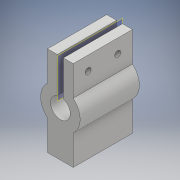
# Autodesk Inventor part: leverClamp
Saved by Autodesk Inventor 2018 (Build 220112000, 112)
## iProperties
Created: 2017-10-29
Part Number: leverClamp
Material: Generic
Document SubType Name: Modeling
Designer: Prakash
Density: 1 g/cm^3
Appearance: Default
Author: Prakash
Autodesk Inventor part; units mm, degrees
ref_plane "YZ Plane" through (0, 0, 0) normal (1, 0, 0) x (0, 1, 0)
ref_plane "XZ Plane" through (0, 0, 0) normal (0, 1, 0) x (-1, 0, 0)
ref_plane "XY Plane" through (0, 0, 0) normal (0, 0, 1) x (1, 0, 0)
sketch "Sketch1" plane through (0, 0, 0) normal (0, 1, 0) x (-1, 0, 0)
  arc A0 (5, -18) -> (5, -27.5394) centre (6.5, -22.7697) ccw
  line L0 (5, 0) -> (5, -18)
  line L1 (5, -27.5394) -> (5, -45.5394)
  line L2 (5, -18) -> (5, -27.5394) construction
  line L3 (5, -22.7697) -> (6.5, -22.7697) construction
  arc A1 (0, -15.1704) -> (0, -30.369) centre (6.5, -22.7697) ccw
  line L4 (0, 0) -> (0, -15.1704)
  line L5 (0, -30.369) -> (0, -45.5394)
  line L6 (5, 0) -> (0, 0)
  line L7 (0, -45.5394) -> (5, -45.5394)
  dimension "d0" = 10
  dimension "d1" = 1.5
  dimension "d2" = 5
  dimension "d4" = 5
  dimension "d5" = 18
  constraints: 16 end point, 5 point on circle, 3 coincident, 2 centre point, 2 collinear, 2 equal length, 2 horizontal, 2 vertical, 1 midpoint, 1 parallel
  measures "d0" diameter of A0
  measures "d1" distance of L3.start L3.end
  measures "d2" radial gap between concentric circles of A1 A0
  measures "d4" distance between parallel lines of L0 L4
  measures "d5" distance of L0.start L0.end
extrude "Extrusion1" add sketch "Sketch1" along normal blind 30
sketch "Sketch2" plane through (0, 0, 0) normal (1, 0, 0) x (0, 0, -1)
  line L0 (45.5394, 30) -> (27.5394, 30) projected
  line L1 (38.5394, 30) -> (38.5394, 0)
  line L2 (45.5394, 0) -> (45.5394, 30) projected
  line L3 (18, 30) -> (0, 30) projected
  line L4 (7, 30) -> (7, 0)
  line L5 (0, 0) -> (0, 30) projected
  line L6 (0, 0) -> (15.1704, 0) projected
  line L7 (30.369, 0) -> (45.5394, 0) projected
  point P0 (38.5394, 22.5)
  point P1 (38.5394, 7.5)
  point P2 (7, 22.5)
  point P3 (7, 7.5)
  dimension "d8" = 7
  dimension "d9" = 7
  dimension "d10" = 7.5
  dimension "d11" = 7.5
  dimension "d12" = 7.5
  dimension "d13" = 7.5
  dimension "d14" = 30
  dimension "d15" = 30
  constraints: 6 point on line, 4 end point, 2 vertical
  measures "d8" distance between parallel lines of L2 L1
  measures "d9" distance between parallel lines of L5 L4
  measures "d10" distance from line of L3 point (7, 22.5)
  measures "d11" distance from line of L6 point (7, 7.5)
  measures "d12" distance from line of L0 point (38.539, 22.5)
  measures "d13" distance from line of L7 point (38.539, 7.5)
  measures "d14" distance from line of L1.end L0
  measures "d15" distance from line of L4.end L0
hole "Hole1" at (0, 22.5, -7) at (0, 7.5, -7) direction (-1, 0, 0) diameter 3 end through all
ref_plane "Work Plane1" through (-6.5, 0, -18) normal (-1, 0, 0) x (0, 0, 1)
mirror "Mirror1" about plane through (-6.5, 0, -18) normal (-1, 0, 0) of "Extrusion1", "Hole1"
sketch "Sketch4" plane through (0, 30, 0) normal (0, 1, 0) x (1, 0, 0)
  arc A0 (-5, 18) -> (-5, 27.5394) centre (-6.5, 22.7697) ccw projected
  arc A1 (-8, 27.5394) -> (-8, 18) centre (-6.5, 22.7697) ccw projected
  arc A2 (-5, 27.5394) -> (-8, 27.5394) centre (-6.5, 22.7697) ccw
  line L0 (-5, 45.5394) -> (-5, 27.5394) projected
  line L1 (-8, 45.5394) -> (-8, 27.5394) projected
  line L2 (-5, 45.5394) -> (-8, 45.5394)
  line L3 (-5, 27.5394) -> (-5, 45.5394)
  line L4 (-8, 45.5394) -> (-8, 27.5394)
  point P0 (0, 0)
  constraints: 6 end point, 2 collinear, 2 point on circle, 1 centre point, 1 coincident, 1 concentric, 1 perpendicular
extrude "Extrusion2" add sketch "Sketch4" against normal up to surface (30 mm away)
equation "\"d11\" = d10"
equation "\"d12\" = d10"
equation "\"d13\" = d10"
body "Solid1"
